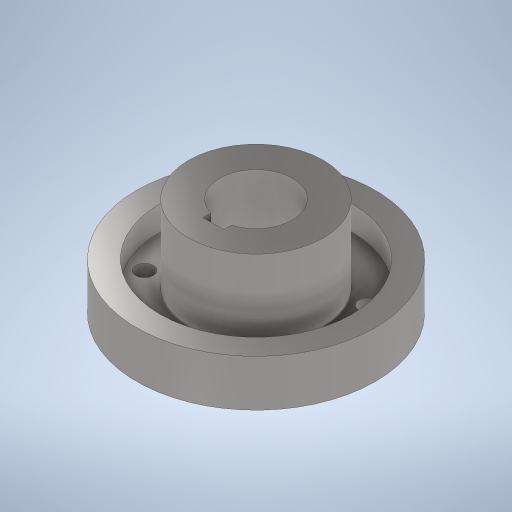
# Autodesk Inventor part: projektspojkas2v1
Saved by Autodesk Inventor 2023 (Build 270158000, 158)
## iProperties
Created: 2023-05-05
Part Number: projektspojkas2v1
Material: Sedá litina
Document SubType Name: Modeling
Designer: S21Suk
Density: 7.85 g/cm^3
Appearance: Pololeštěná
Description: Kotoučová spojka
Polotovar: Odlitek
Author: S21Suk
Autodesk Inventor part; units mm, degrees
ref_plane "YZ Plane" through (0, 0, 0) normal (1, 0, 0) x (0, 1, 0)
ref_plane "XZ Plane" through (0, 0, 0) normal (0, 1, 0) x (-1, 0, 0)
ref_plane "XY Plane" through (0, 0, 0) normal (0, 0, 1) x (1, 0, 0)
sketch "Náčrt1" plane through (0, 0, 0) normal (0, 1, 0) x (-1, 0, 0)
  circle A0 centre (0, 0) radius 115
  circle A1 centre (0, 0) radius 92.5
  circle A2 centre (0, 0) radius 35
  circle A3 centre (0, 0) radius 65
  dimension "d0" = 230
  dimension "d1" = 185
  dimension "d2" = 70
  dimension "d3" = 130
  constraints: 4 centre point, 4 coincident
  measures "d0" diameter of A0
  measures "d1" diameter of A1
  measures "d2" diameter of A2
  measures "d3" diameter of A3
extrude "Vysunutí1" add sketch "Náčrt1" along normal blind 95 contours A3
extrude "Vysunutí2" add sketch "Náčrt1" along normal blind 21 contours A1
extrude "Vysunutí3" add sketch "Náčrt1" along normal blind 45 contours A0
sketch "Náčrt2" plane through (0, 21, 0) normal (0, 1, 0) x (1, 0, 0)
  circle A0 centre (0, 0) radius 65 construction
  line L0 (0, -65) -> (0, -92.5) construction
  circle A1 centre (0, 0) radius 92.5 construction
  circle A2 centre (0, -78.75) radius 8.5
  circle A3 centre (68.1995, -39.375) radius 8.5
  circle A4 centre (68.1995, 39.375) radius 8.5
  circle A5 centre (0, 78.75) radius 8.5
  circle A6 centre (-68.1995, 39.375) radius 8.5
  circle A7 centre (-68.1995, -39.375) radius 8.5
  dimension "d10" = 27.5
  dimension "d11" = 17
  dimension "d14" = 360
  constraints: 6 centre point, 2 end point, 2 vertical alignment, 1 midpoint, 1 vertical, 15 other
  measures "d10" distance of L0.start L0.end
  measures "d11" diameter of A2
extrude "Vysunutí4" cut sketch "Náčrt2" against normal through all
sketch "Náčrt3" plane through (0, 0, 0) normal (0, -1, 0) x (1, 0, 0)
  line L0 (-10, 41) -> (10, 41)
  line L1 (10, 41) -> (10, 29)
  line L2 (10, 29) -> (-10, 29)
  line L3 (-10, 29) -> (-10, 41)
  circle A0 centre (0, 0) radius 35 projected
  line L4 (-10, 41) -> (10, 29) construction
  line L5 (10, 41) -> (-10, 29) construction
  point P0 (0, 35)
  point P1 (0, 29)
  dimension "d18" = 20
  dimension "d19" = 12
  dimension "d20" = 29
  constraints: 12 end point, 3 midpoint, 2 parallel, 1 horizontal, 1 perpendicular, 1 vertical alignment, 1 other
  measures "d18" distance of L1.end L2.end
  measures "d19" distance between parallel lines of L0 L2
  measures "d20" distance of point (0, 0) point (0, 29)
extrude "Vysunutí5" cut sketch "Náčrt3" against normal through all contours L0 L1 A0 L3 | A0 L1 L2 L3 picked at (1.1251, 30.9456)
